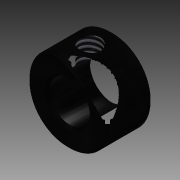
# Autodesk Inventor part: Misc_ShaftCollar_Ruland_SC-4-F
Saved by Autodesk Inventor 2014 (Build 180170000, 170)
## iProperties
Category: Miscellaneous
Company: Autodesk Inc.
Created: 2012-12-03
Part Number: Misc_ShaftCollar_Ruland_SC-4-F
Document SubType Name: Modeling
Designer: Autodesk Inc.
Density: 7.87 g/cm^3
Material: Steel, Carbon
Appearance: Smooth - Black
Author: Autodesk Inc.
Autodesk Inventor part; units mm, degrees
note: some values were not read from the file. Chosen so that the rebuilt part matches the saved one: direction of "Hole1".
ref_plane "YZ Plane" through (0, 0, 0) normal (1, 0, 0) x (0, 1, 0)
ref_plane "XY Plane" through (0, 0, 0) normal (0, 0, 1) x (1, 0, 0)
sketch "Sketch1" plane through (0, 0, 0) normal (0, 0, 1) x (1, 0, 0)
  circle A0 centre (0, 0) radius 6.35
  dimension "d0" = 12.7
  constraints: 1 centre point, 1 coincident
  measures "d0" diameter of A0
extrude "Extrusion1" add sketch "Sketch1" against normal blind 7.1374
sketch "Sketch2" plane through (0, 0, 0) normal (0, 0, 1) x (1, 0, 0)
  circle A0 centre (0, 0) radius 6.35 projected
  circle A1 centre (0, 0) radius 3.175
  dimension "d3" = 6.35
  constraints: 1 centre point, 1 coincident
  measures "d3" diameter of A1
extrude "Extrusion2" cut sketch "Sketch2" against normal up to next contours A1
chamfer "Chamfer1" distance 0.3969 angle 45 4 edges at (-6.35, 0, 0) (-6.35, 0, -7.1374) (-3.175, 0, 0) (-3.175, 0, -7.1374)
ref_plane "Work Plane1" through (0, 6.35, 0) normal (0, 1, 0) x (-1, 0, 0)
sketch "Sketch3" plane through (0, 6.35, 0) normal (0, 1, 0) x (-1, 0, 0)
  line L0 (5.9531, -7.1374) -> (-5.9531, -7.1374) projected
  line L1 (6.35, -0.3969) -> (6.35, -6.7405) projected
  point P0 (0, 0)
  point P1 (0, -3.5687)
hole "Hole1" at (0, 6.35, -3.5687) direction (0, -1, 0) diameter 3.302 end up to surface thread size "8-32 UNC" class "2B" standard "ANSI Unified Screw Threads"
body "Solid1"
